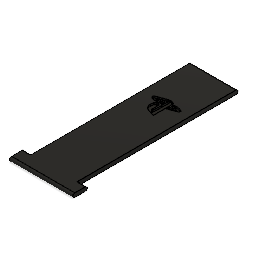
VitaStand v1 (Autodesk Fusion 360 design; units mm, degrees)
Autodesk Fusion 360 part; units mm, degrees
sketch "Sketch1" plane through (0, 0, 0) normal (0, 1, 0) x (1, 0, 0)
  line L0 (-29.9142, 7) -> (-29.9142, 0)
  line L1 (-29.9142, 0) -> (0, 0)
  line L2 (0, 0) -> (0, 7)
  line L3 (-4, 7) -> (-4, 82.0708)
  line L4 (-4, 82.0708) -> (-25.9976, 82.0708)
  line L5 (-25.9976, 82.0708) -> (-25.9976, 7)
  line L6 (0, 7) -> (-4, 7)
  line L7 (-25.9976, 7) -> (-29.9142, 7)
extrude "Extrude1" add sketch "Sketch1" along normal blind 2
fillet "Fillet1" radius 1 2 edges at (-14.9571, 2, 0) (-14.9571, 0, 0)
fillet "Fillet2" radius 1 2 edges at (-14.9988, 2, -82.0708) (-14.9988, 0, -82.0708)
fillet "Fillet3" radius 1 2 edges at (-2, 0, -7) (-2, 2, -7)
fillet "Fillet4" radius 1 2 edges at (-27.9559, 0, -7) (-27.9559, 2, -7)
sketch "Sketch2" plane through (0, 2, 0) normal (0, 1, 0) x (-1, 0, 0)
  line L0 (25.9976, -6) -> (29.9142, -6)
  line L1 (29.9142, -6) -> (29.9142, -1)
  line L2 (29.9142, -1) -> (0, -1)
  line L3 (0, -1) -> (0, -6)
  line L4 (0, -6) -> (4, -6)
  line L5 (4, -6) -> (4, -81.0708)
  line L6 (4, -81.0708) -> (25.9976, -81.0708)
  line L7 (25.9976, -81.0708) -> (25.9976, -6)
  line L8 (13.1427, -55.9691) -> (13.1729, -60.7147)
  line L9 (13.1729, -60.7147) -> (14.0777, -61.0465)
  spline S0 degree 3 poles (14.0777, -61.0464) (14.5804, -61.2274) (15.0429, -61.3782) (15.1033, -61.3782) knots 0 0 0 0 1 1 1 1
  spline S1 degree 3 poles (15.1033, -61.3782) (15.2038, -61.3883) (15.234, -60.4432) (15.2541, -57.1454) knots 0 0 0 0 1 1 1 1
  spline S2 degree 3 poles (15.2541, -57.1454) (15.2842, -53.1238) (15.2943, -52.8925) (15.4652, -52.8624) knots 0 0 0 0 1 1 1 1
  spline S3 degree 3 poles (15.4652, -52.8624) (15.5657, -52.8422) (15.7367, -52.9026) (15.8473, -53.0031) knots 0 0 0 0 1 1 1 1
  spline S4 degree 3 poles (15.8473, -53.0031) (16.0182, -53.164) (16.0383, -53.3248) (16.0383, -55.024) knots 0 0 0 0 1 1 1 1
  line L10 (16.0383, -55.024) -> (16.0383, -56.874)
  line L11 (16.0383, -56.874) -> (16.3902, -57.0248)
  spline S5 degree 3 poles (16.3902, -57.0248) (17.1443, -57.3365) (17.8179, -57.0952) (18.1698, -56.3813) knots 0 0 0 0 1 1 1 1
  spline S6 degree 3 poles (18.1698, -56.3813) (18.3608, -55.9892) (18.401, -55.7479) (18.401, -55.0039) knots 0 0 0 0 1 1 1 1
  spline S7 degree 3 poles (18.401, -55.0039) (18.401, -54.1895) (18.3709, -54.0488) (18.0994, -53.5561) knots 0 0 0 0 1 1 1 1
  spline S8 degree 3 poles (18.0994, -53.5561) (17.8179, -53.0333) (17.3453, -52.611) (16.7119, -52.2792) knots 0 0 0 0 1 1 1 1
  spline S9 degree 3 poles (16.7119, -52.2792) (16.4505, -52.1385) (13.394, -51.2336) (13.203, -51.2336) knots 0 0 0 0 1 1 1 1
  spline S10 degree 3 poles (13.203, -51.2336) (13.1527, -51.2336) (13.1326, -53.3651) (13.1427, -55.9691) knots 0 0 0 0 1 1 1 1
  spline S11 degree 3 poles (10.8604, -57.6079) (8.9602, -58.3117) (8.6284, -58.4625) (8.3569, -58.7642) knots 0 0 0 0 1 1 1 1
  spline S12 degree 3 poles (8.3569, -58.7642) (8.1156, -59.0256) (8.2061, -59.4177) (8.558, -59.6389) knots 0 0 0 0 1 1 1 1
  spline S13 degree 3 poles (8.558, -59.6389) (9.1914, -60.0611) (11.0112, -60.3728) (12.0568, -60.2421) knots 0 0 0 0 1 1 1 1
  line L12 (12.0568, -60.2421) -> (12.6199, -60.1717)
  line L13 (12.6199, -60.1717) -> (12.6199, -59.6188)
  spline S14 degree 3 poles (12.6199, -59.6188) (12.6199, -59.3171) (12.5897, -59.0758) (12.5495, -59.0758) knots 0 0 0 0 1 1 1 1
  spline S15 degree 3 poles (12.5495, -59.0758) (12.5193, -59.0758) (12.1473, -59.1965) (11.7351, -59.3372) knots 0 0 0 0 1 1 1 1
  spline S16 degree 3 poles (11.7351, -59.3372) (11.1821, -59.5283) (10.8906, -59.5785) (10.5889, -59.5283) knots 0 0 0 0 1 1 1 1
  spline S17 degree 3 poles (10.5889, -59.5283) (9.9254, -59.4076) (10.1466, -59.1965) (11.4636, -58.6837) knots 0 0 0 0 1 1 1 1
  line L14 (11.4636, -58.6837) -> (12.6701, -58.2212)
  line L15 (12.6701, -58.2212) -> (12.7003, -57.5878)
  spline S18 degree 3 poles (12.7003, -57.5878) (12.7204, -57.246) (12.6903, -56.9645) (12.65, -56.9745) knots 0 0 0 0 1 1 1 1
  spline S19 degree 3 poles (12.65, -56.9745) (12.6098, -56.9745) (11.8055, -57.2661) (10.8604, -57.6079) knots 0 0 0 0 1 1 1 1
  spline S20 degree 3 poles (16.9934, -57.5778) (16.722, -57.618) (16.2997, -57.7085) (16.0685, -57.7788) knots 0 0 0 0 1 1 1 1
  line L16 (16.0685, -57.7788) -> (15.6361, -57.8995)
  line L17 (15.6361, -57.8995) -> (15.6361, -58.543)
  spline S21 degree 3 poles (15.6361, -58.543) (15.6361, -59.1261) (15.6562, -59.1965) (15.8171, -59.1462) knots 0 0 0 0 1 1 1 1
  spline S22 degree 3 poles (15.8171, -59.1462) (15.9076, -59.1161) (16.4606, -58.925) (17.0437, -58.7239) knots 0 0 0 0 1 1 1 1
  spline S23 degree 3 poles (17.0437, -58.7239) (17.6269, -58.5229) (18.2804, -58.3419) (18.5116, -58.3017) knots 0 0 0 0 1 1 1 1
  spline S24 degree 3 poles (18.5116, -58.3017) (18.9942, -58.2413) (19.4265, -58.4123) (19.2657, -58.6133) knots 0 0 0 0 1 1 1 1
  spline S25 degree 3 poles (19.2657, -58.6133) (19.2054, -58.6837) (18.3709, -59.0256) (17.3956, -59.3775) knots 0 0 0 0 1 1 1 1
  line L18 (17.3956, -59.3775) -> (15.6361, -60.0109)
  line L19 (15.6361, -60.0109) -> (15.6361, -60.6342)
  line L20 (15.6361, -60.6342) -> (15.6361, -61.2576)
  line L21 (15.6361, -61.2576) -> (18.1095, -60.3728)
  spline S26 degree 3 poles (18.1095, -60.3728) (20.6129, -59.4679) (21.1056, -59.2367) (21.2162, -58.8647) knots 0 0 0 0 1 1 1 1
  spline S27 degree 3 poles (21.2162, -58.8647) (21.4977, -58) (19.0043, -57.2359) (16.9934, -57.5778) knots 0 0 0 0 1 1 1 1
extrude "Extrude2" cut sketch "Sketch2" along normal mid plane 1.6 contours L8 L9 S0 S1 S2 S3 S4 L10 L11 S5 S6 S7 S8 S9 S10 | S11 S12 S13 L12 L13 S14 S15 S16 S17 L14 L15 S18 S19 | S20 L16 L17 S21 S22 S23 S24 S25 L18 L19 L20 L21 S26 S27
